Autodesk Fusion 360 part; units mm, degrees
(part 4 of 9)
  spline S95 degree 3 poles (-31.9349, 64.8889) (-32.1312, 64.9819) (-32.4392, 65.0284) (-32.8599, 65.0284) knots 0 0 0 0 1 1 1 1
  line L121 (-32.8599, 65.0284) -> (-35.2008, 65.0284)
  line L122 (-35.2008, 65.0284) -> (-35.2008, 61.7728)
  line L123 (-35.2008, 61.7728) -> (-36.2292, 61.7728)
  line L124 (-36.2292, 61.7728) -> (-36.2292, 69.3641)
  line L125 (-13.5711, 69.3641) -> (-13.5711, 68.4598)
  line L126 (-13.5711, 68.4598) -> (-16.1291, 68.4598)
  line L127 (-16.1291, 68.4598) -> (-16.1291, 61.7728)
  line L128 (-16.1291, 61.7728) -> (-17.173, 61.7728)
  line L129 (-17.173, 61.7728) -> (-17.173, 68.4598)
  line L130 (-17.173, 68.4598) -> (-19.7309, 68.4598)
  line L131 (-19.7309, 68.4598) -> (-19.7309, 69.3641)
  line L132 (-19.7309, 69.3641) -> (-13.5711, 69.3641)
  line L133 (-1.8995, 69.3641) -> (-1.8995, 64.6719)
  spline S96 degree 3 poles (-1.8995, 64.6719) (-1.8995, 64.121) (-1.7961, 63.6621) (-1.5894, 63.2973) knots 0 0 0 0 1 1 1 1
  spline S97 degree 3 poles (-1.5894, 63.2973) (-1.2825, 62.7464) (-0.7657, 62.4705) (-0.0391, 62.4705) knots 0 0 0 0 1 1 1 1
  spline S98 degree 3 poles (-0.0391, 62.4705) (0.8321, 62.4705) (1.4254, 62.7681) (1.7385, 63.3645) knots 0 0 0 0 1 1 1 1
  spline S99 degree 3 poles (1.7385, 63.3645) (1.907, 63.688) (1.9918, 64.1241) (1.9918, 64.6719) knots 0 0 0 0 1 1 1 1
  line L134 (1.9918, 64.6719) -> (1.9918, 69.3641)
  line L135 (1.9918, 69.3641) -> (3.0356, 69.3641)
  line L136 (3.0356, 69.3641) -> (3.0356, 65.1008)
  spline S100 degree 3 poles (3.0356, 65.1008) (3.0356, 64.1675) (2.9095, 63.4492) (2.6584, 62.9459) knots 0 0 0 0 1 1 1 1
  spline S101 degree 3 poles (2.6584, 62.9459) (2.1964, 62.0291) (1.3251, 61.5713) (0.0436, 61.5713) knots 0 0 0 0 1 1 1 1
  spline S102 degree 3 poles (0.0436, 61.5713) (-1.238, 61.5713) (-2.1083, 62.0291) (-2.5661, 62.9459) knots 0 0 0 0 1 1 1 1
  spline S103 degree 3 poles (-2.5661, 62.9459) (-2.8173, 63.4492) (-2.9433, 64.1675) (-2.9433, 65.1008) knots 0 0 0 0 1 1 1 1
  line L137 (-2.9433, 65.1008) -> (-2.9433, 69.3641)
  line L138 (-2.9433, 69.3641) -> (-1.8995, 69.3641)
  line L139 (13.6531, 69.3641) -> (14.8675, 69.3641)
  line L140 (14.8675, 69.3641) -> (18.7018, 63.2146)
  line L141 (18.7018, 63.2146) -> (18.7018, 69.3641)
  line L142 (18.7018, 69.3641) -> (19.6785, 69.3641)
  line L143 (19.6785, 69.3641) -> (19.6785, 61.7728)
  line L144 (19.6785, 61.7728) -> (18.5261, 61.7728)
  line L145 (18.5261, 61.7728) -> (14.6349, 67.9172)
  line L146 (14.6349, 67.9172) -> (14.6349, 61.7728)
  line L147 (14.6349, 61.7728) -> (13.6531, 61.7728)
  line L148 (13.6531, 61.7728) -> (13.6531, 69.3641)
  line L149 (31.0091, 69.3641) -> (36.2749, 69.3641)
  line L150 (36.2749, 69.3641) -> (36.2749, 68.4339)
  line L151 (36.2749, 68.4339) -> (32.0375, 68.4339)
  line L152 (32.0375, 68.4339) -> (32.0375, 66.1292)
  line L153 (32.0375, 66.1292) -> (35.7633, 66.1292)
  line L154 (35.7633, 66.1292) -> (35.7633, 65.2248)
  line L155 (35.7633, 65.2248) -> (32.0375, 65.2248)
  line L156 (32.0375, 65.2248) -> (32.0375, 61.7728)
  line L157 (32.0375, 61.7728) -> (31.0091, 61.7728)
  line L158 (31.0091, 61.7728) -> (31.0091, 69.3641)
  line L159 (47.0164, 62.6255) -> (51.6724, 68.4598)
  line L160 (51.6724, 68.4598) -> (47.3575, 68.4598)
  line L161 (47.3575, 68.4598) -> (47.3575, 69.3641)
  line L162 (47.3575, 69.3641) -> (52.9954, 69.3641)
  line L163 (52.9954, 69.3641) -> (52.9954, 68.4804)
  line L164 (52.9954, 68.4804) -> (48.3135, 62.6772)
  line L165 (48.3135, 62.6772) -> (52.9954, 62.6772)
  line L166 (52.9954, 62.6772) -> (52.9954, 61.7728)
  line L167 (52.9954, 61.7728) -> (47.0164, 61.7728)
  line L168 (47.0164, 61.7728) -> (47.0164, 62.6255)
  line L169 (67.8482, 64.8837) -> (66.6958, 68.2375)
  line L170 (66.6958, 68.2375) -> (65.4711, 64.8837)
  line L171 (65.4711, 64.8837) -> (67.8482, 64.8837)
  line L172 (66.1584, 69.3641) -> (67.3211, 69.3641)
  line L173 (67.3211, 69.3641) -> (70.0755, 61.7728)
  line L174 (70.0755, 61.7728) -> (68.9489, 61.7728)
  line L175 (68.9489, 61.7728) -> (68.1789, 64.0466)
  line L176 (68.1789, 64.0466) -> (65.1765, 64.0466)
  line L177 (65.1765, 64.0466) -> (64.3549, 61.7728)
  line L178 (64.3549, 61.7728) -> (63.3007, 61.7728)
  line L179 (63.3007, 61.7728) -> (66.1584, 69.3641)
  line L180 (67.0576, 71.1624) -> (68.0239, 71.1624)
  line L181 (68.0239, 71.1624) -> (68.0239, 70.0876)
  line L182 (68.0239, 70.0876) -> (67.0576, 70.0876)
  line L183 (67.0576, 70.0876) -> (67.0576, 71.1624)
  line L184 (65.3522, 71.1624) -> (66.3186, 71.1624)
  line L185 (66.3186, 71.1624) -> (66.3186, 70.0876)
  line L186 (66.3186, 70.0876) -> (65.3522, 70.0876)
  line L187 (65.3522, 70.0876) -> (65.3522, 71.1624)
  line L188 (84.517, 64.8837) -> (83.3646, 68.2375)
  line L189 (83.3646, 68.2375) -> (82.1398, 64.8837)
  line L190 (82.1398, 64.8837) -> (84.517, 64.8837)
  line L191 (82.8271, 69.3641) -> (83.9899, 69.3641)
  line L192 (83.9899, 69.3641) -> (86.7442, 61.7728)
  line L193 (86.7442, 61.7728) -> (85.6177, 61.7728)
  line L194 (85.6177, 61.7728) -> (84.8477, 64.0466)
  line L195 (84.8477, 64.0466) -> (81.8453, 64.0466)
  line L196 (81.8453, 64.0466) -> (81.0236, 61.7728)
  line L197 (81.0236, 61.7728) -> (79.9694, 61.7728)
  line L198 (79.9694, 61.7728) -> (82.8271, 69.3641)
  line L199 (83.7263, 71.1624) -> (84.6927, 71.1624)
  line L200 (84.6927, 71.1624) -> (84.6927, 70.0876)
  line L201 (84.6927, 70.0876) -> (83.7263, 70.0876)
  line L202 (83.7263, 70.0876) -> (83.7263, 71.1624)
  line L203 (82.021, 71.1624) -> (82.9873, 71.1624)
  line L204 (82.9873, 71.1624) -> (82.9873, 70.0876)
  line L205 (82.9873, 70.0876) -> (82.021, 70.0876)
  line L206 (82.021, 70.0876) -> (82.021, 71.1624)
  line L207 (-86.3336, 44.1253) -> (-81.6776, 49.9596)
  line L208 (-81.6776, 49.9596) -> (-85.9925, 49.9596)
  line L209 (-85.9925, 49.9596) -> (-85.9925, 50.8639)
  line L210 (-85.9925, 50.8639) -> (-80.3546, 50.8639)
  line L211 (-80.3546, 50.8639) -> (-80.3546, 49.9803)
  line L212 (-80.3546, 49.9803) -> (-85.0365, 44.177)
  line L213 (-85.0365, 44.177) -> (-80.3546, 44.177)
  line L214 (-80.3546, 44.177) -> (-80.3546, 43.2727)
  line L215 (-80.3546, 43.2727) -> (-86.3336, 43.2727)
  line L216 (-86.3336, 43.2727) -> (-86.3336, 44.1253)
  line L217 (-70.3615, 50.8639) -> (-68.93, 44.6886)
  line L218 (-68.93, 44.6886) -> (-67.2144, 50.8639)
  line L219 (-67.2144, 50.8639) -> (-66.0981, 50.8639)
  line L220 (-66.0981, 50.8639) -> (-64.3825, 44.6886)
  line L221 (-64.3825, 44.6886) -> (-62.951, 50.8639)
  line L222 (-62.951, 50.8639) -> (-61.8245, 50.8639)
  line L223 (-61.8245, 50.8639) -> (-63.8192, 43.2727)
  line L224 (-63.8192, 43.2727) -> (-64.8993, 43.2727)
  line L225 (-64.8993, 43.2727) -> (-66.6511, 49.5669)
  line L226 (-66.6511, 49.5669) -> (-68.4132, 43.2727)
  line L227 (-68.4132, 43.2727) -> (-69.4933, 43.2727)
  line L228 (-69.4933, 43.2727) -> (-71.4777, 50.8639)
  line L229 (-71.4777, 50.8639) -> (-70.3615, 50.8639)
  line L230 (-48.833, 46.3836) -> (-49.9854, 49.7374)
  line L231 (-49.9854, 49.7374) -> (-51.2102, 46.3836)
  line L232 (-51.2102, 46.3836) -> (-48.833, 46.3836)
  line L233 (-50.5229, 50.8639) -> (-49.3601, 50.8639)
  line L234 (-49.3601, 50.8639) -> (-46.6058, 43.2727)
  line L235 (-46.6058, 43.2727) -> (-47.7323, 43.2727)
  line L236 (-47.7323, 43.2727) -> (-48.5023, 45.5464)
  line L237 (-48.5023, 45.5464) -> (-51.5047, 45.5464)
  line L238 (-51.5047, 45.5464) -> (-52.3264, 43.2727)
  line L239 (-52.3264, 43.2727) -> (-53.3806, 43.2727)
  line L240 (-53.3806, 43.2727) -> (-50.5229, 50.8639)
  line L241 (-49.6237, 52.6623) -> (-48.6573, 52.6623)
  line L242 (-48.6573, 52.6623) -> (-48.6573, 51.5874)
  line L243 (-48.6573, 51.5874) -> (-49.6237, 51.5874)
  line L244 (-49.6237, 51.5874) -> (-49.6237, 52.6623)
  line L245 (-51.329, 52.6623) -> (-50.3627, 52.6623)
  line L246 (-50.3627, 52.6623) -> (-50.3627, 51.5874)
  line L247 (-50.3627, 51.5874) -> (-51.329, 51.5874)
  line L248 (-51.329, 51.5874) -> (-51.329, 52.6623)
  line L249 (-36.3532, 50.8639) -> (-35.1388, 50.8639)
  line L250 (-35.1388, 50.8639) -> (-31.3044, 44.7144)
  line L251 (-31.3044, 44.7144) -> (-31.3044, 50.8639)
  line L252 (-31.3044, 50.8639) -> (-30.3277, 50.8639)
  line L253 (-30.3277, 50.8639) -> (-30.3277, 43.2727)
  line L254 (-30.3277, 43.2727) -> (-31.4801, 43.2727)
  line L255 (-31.4801, 43.2727) -> (-35.3713, 49.417)
  line L256 (-35.3713, 49.417) -> (-35.3713, 43.2727)
  line L257 (-35.3713, 43.2727) -> (-36.3532, 43.2727)
  line L258 (-36.3532, 43.2727) -> (-36.3532, 50.8639)
  line L259 (-19.6586, 44.1253) -> (-15.0026, 49.9596)
  line L260 (-15.0026, 49.9596) -> (-19.3175, 49.9596)
  line L261 (-19.3175, 49.9596) -> (-19.3175, 50.8639)
  line L262 (-19.3175, 50.8639) -> (-13.6796, 50.8639)
  line L263 (-13.6796, 50.8639) -> (-13.6796, 49.9803)
  line L264 (-13.6796, 49.9803) -> (-18.3615, 44.177)
  line L265 (-18.3615, 44.177) -> (-13.6796, 44.177)
  line L266 (-13.6796, 44.177) -> (-13.6796, 43.2727)
  line L267 (-13.6796, 43.2727) -> (-19.6586, 43.2727)
  line L268 (-19.6586, 43.2727) -> (-19.6586, 44.1253)
  spline S104 degree 3 poles (-0.0278, 51.0603) (0.6854, 51.0603) (1.3024, 50.9228) (1.8223, 50.6469) knots 0 0 0 0 1 1 1 1
  spline S105 degree 3 poles (1.8223, 50.6469) (2.5767, 50.251) (3.0387, 49.5565) (3.2072, 48.5643) knots 0 0 0 0 1 1 1 1
  line L269 (3.2072, 48.5643) -> (2.1892, 48.5643)
  spline S106 degree 3 poles (2.1892, 48.5643) (2.0651, 49.1193) (1.8088, 49.5234) (1.4192, 49.7756) knots 0 0 0 0 1 1 1 1
  spline S107 degree 3 poles (1.4192, 49.7756) (1.0295, 50.0288) (0.5386, 50.156) (-0.0536, 50.156) knots 0 0 0 0 1 1 1 1
  spline S108 degree 3 poles (-0.0536, 50.156) (-0.7564, 50.156) (-1.3476, 49.8924) (-1.8292, 49.3653) knots 0 0 0 0 1 1 1 1
  spline S109 degree 3 poles (-1.8292, 49.3653) (-2.3098, 48.8382) (-2.5496, 48.0527) (-2.5496, 47.0089) knots 0 0 0 0 1 1 1 1
  spline S110 degree 3 poles (-2.5496, 47.0089) (-2.5496, 46.1066) (-2.3511, 45.3718) (-1.9553, 44.8044) knots 0 0 0 0 1 1 1 1
  spline S111 degree 3 poles (-1.9553, 44.8044) (-1.5594, 44.238) (-0.9135, 43.9548) (-0.0174, 43.9548) knots 0 0 0 0 1 1 1 1
  spline S112 degree 3 poles (-0.0174, 43.9548) (0.6678, 43.9548) (1.2362, 44.1532) (1.6848, 44.5522) knots 0 0 0 0 1 1 1 1
  spline S113 degree 3 poles (1.6848, 44.5522) (2.1344, 44.9501) (2.3649, 45.5929) (2.3752, 46.4818) knots 0 0 0 0 1 1 1 1
  line L270 (2.3752, 46.4818) -> (-0.0019, 46.4818)
  line L271 (-0.0019, 46.4818) -> (-0.0019, 47.3344)
  line L272 (-0.0019, 47.3344) -> (3.3312, 47.3344)
  line L273 (3.3312, 47.3344) -> (3.3312, 43.2727)
  line L274 (3.3312, 43.2727) -> (2.6698, 43.2727)
  line L275 (2.6698, 43.2727) -> (2.4217, 44.2493)
  spline S114 degree 3 poles (2.4217, 44.2493) (2.0734, 43.8669) (1.7654, 43.6013) (1.4967, 43.4535) knots 0 0 0 0 1 1 1 1
  spline S115 degree 3 poles (1.4967, 43.4535) (1.045, 43.1983) (0.4714, 43.0711) (-0.2241, 43.0711) knots 0 0 0 0 1 1 1 1
  spline S116 degree 3 poles (-0.2241, 43.0711) (-1.1233, 43.0711) (-1.8964, 43.3626) (-2.5444, 43.9445) knots 0 0 0 0 1 1 1 1
  spline S117 degree 3 poles (-2.5444, 43.9445) (-3.2503, 44.6752) (-3.6038, 45.6777) (-3.6038, 46.952) knots 0 0 0 0 1 1 1 1
  spline S118 degree 3 poles (-3.6038, 46.952) (-3.6038, 48.2233) (-3.2596, 49.2341) (-2.5702, 49.9854) knots 0 0 0 0 1 1 1 1
  spline S119 degree 3 poles (-2.5702, 49.9854) (-1.916, 50.7017) (-1.0685, 51.0603) (-0.0278, 51.0603) knots 0 0 0 0 1 1 1 1
  spline S120 degree 3 poles (14.6173, 45.7221) (14.6411, 45.2911) (14.7434, 44.9418) (14.9222, 44.6731) knots 0 0 0 0 1 1 1 1
  spline S121 degree 3 poles (14.9222, 44.6731) (15.2633, 44.1698) (15.8648, 43.9186) (16.7257, 43.9186) knots 0 0 0 0 1 1 1 1
  spline S122 degree 3 poles (16.7257, 43.9186) (17.1112, 43.9186) (17.4626, 43.9734) (17.7799, 44.084) knots 0 0 0 0 1 1 1 1
  spline S123 degree 3 poles (17.7799, 44.084) (18.3928, 44.2979) (18.6998, 44.6803) (18.6998, 45.2312) knots 0 0 0 0 1 1 1 1
  spline S124 degree 3 poles (18.6998, 45.2312) (18.6998, 45.6446) (18.5706, 45.9392) (18.3122, 46.1149) knots 0 0 0 0 1 1 1 1
  spline S125 degree 3 poles (18.3122, 46.1149) (18.0507, 46.2875) (17.6404, 46.4373) (17.0823, 46.5645) knots 0 0 0 0 1 1 1 1
  line L276 (17.0823, 46.5645) -> (16.0539, 46.797)
  spline S126 degree 3 poles (16.0539, 46.797) (15.3822, 46.9489) (14.9067, 47.1153) (14.6277, 47.2983) knots 0 0 0 0 1 1 1 1
  spline S127 degree 3 poles (14.6277, 47.2983) (14.145, 47.6156) (13.9042, 48.0889) (13.9042, 48.7194) knots 0 0 0 0 1 1 1 1
  spline S128 degree 3 poles (13.9042, 48.7194) (13.9042, 49.4015) (14.1399, 49.9617) (14.6122, 50.3988) knots 0 0 0 0 1 1 1 1
  spline S129 degree 3 poles (14.6122, 50.3988) (15.0845, 50.836) (15.7522, 51.0551) (16.6172, 51.0551) knots 0 0 0 0 1 1 1 1
  spline S130 degree 3 poles (16.6172, 51.0551) (17.413, 51.0551) (18.089, 50.8629) (18.646, 50.4784) knots 0 0 0 0 1 1 1 1
  spline S131 degree 3 poles (18.646, 50.4784) (19.2021, 50.095) (19.4801, 49.4811) (19.4801, 48.6367) knots 0 0 0 0 1 1 1 1
  line L277 (19.4801, 48.6367) -> (18.5137, 48.6367)
  spline S132 degree 3 poles (18.5137, 48.6367) (18.4621, 49.0429) (18.3515, 49.355) (18.183, 49.572) knots 0 0 0 0 1 1 1 1
  spline S133 degree 3 poles (18.183, 49.572) (17.8699, 49.9679) (17.3376, 50.1663) (16.5862, 50.1663) knots 0 0 0 0 1 1 1 1
  spline S134 degree 3 poles (16.5862, 50.1663) (15.9795, 50.1663) (15.5444, 50.0392) (15.2788, 49.7839) knots 0 0 0 0 1 1 1 1
  spline S135 degree 3 poles (15.2788, 49.7839) (15.0132, 49.5286) (14.8809, 49.233) (14.8809, 48.8951) knots 0 0 0 0 1 1 1 1
  spline S136 degree 3 poles (14.8809, 48.8951) (14.8809, 48.523) (15.0359, 48.2512) (15.346, 48.0786) knots 0 0 0 0 1 1 1 1
  spline S137 degree 3 poles (15.346, 48.0786) (15.5496, 47.968) (16.0095, 47.8305) (16.7257, 47.6652) knots 0 0 0 0 1 1 1 1
  line L278 (16.7257, 47.6652) -> (17.7903, 47.4223)
  spline S138 degree 3 poles (17.7903, 47.4223) (18.3039, 47.3055) (18.6998, 47.1453) (18.9788, 46.9417) knots 0 0 0 0 1 1 1 1
  spline S139 degree 3 poles (18.9788, 46.9417) (19.4615, 46.5872) (19.7023, 46.0715) (19.7023, 45.3966) knots 0 0 0 0 1 1 1 1
  spline S140 degree 3 poles (19.7023, 45.3966) (19.7023, 44.5563) (19.3964, 43.9548) (18.7845, 43.5931) knots 0 0 0 0 1 1 1 1
  spline S141 degree 3 poles (18.7845, 43.5931) (18.1737, 43.2313) (17.4626, 43.0505) (16.6534, 43.0505) knots 0 0 0 0 1 1 1 1
  spline S142 degree 3 poles (16.6534, 43.0505) (15.7098, 43.0505) (14.9708, 43.2913) (14.4365, 43.7739) knots 0 0 0 0 1 1 1 1
  spline S143 degree 3 poles (14.4365, 43.7739) (13.9021, 44.2524) (13.6407, 44.9025) (13.651, 45.7221) knots 0 0 0 0 1 1 1 1
  line L279 (13.651, 45.7221) -> (14.6173, 45.7221)
  line L280 (30.7125, 50.8639) -> (36.247, 50.8639)
  line L281 (36.247, 50.8639) -> (36.247, 49.9338)
  line L282 (36.247, 49.9338) -> (31.715, 49.9338)
  line L283 (31.715, 49.9338) -> (31.715, 47.629)
  line L284 (31.715, 47.629) -> (35.906, 47.629)
  line L285 (35.906, 47.629) -> (35.906, 46.7505)
  line L286 (35.906, 46.7505) -> (31.715, 46.7505)
  line L287 (31.715, 46.7505) -> (31.715, 44.177)
  line L288 (31.715, 44.177) -> (36.3245, 44.177)
  line L289 (36.3245, 44.177) -> (36.3245, 43.2727)
  line L290 (36.3245, 43.2727) -> (30.7125, 43.2727)
  line L291 (30.7125, 43.2727) -> (30.7125, 50.8639)
  line L292 (47.8825, 50.8639) -> (50.0632, 44.3992)
  line L293 (50.0632, 44.3992) -> (52.2181, 50.8639)
  line L294 (52.2181, 50.8639) -> (53.3705, 50.8639)
  line L295 (53.3705, 50.8639) -> (50.6007, 43.2727)
  line L296 (50.6007, 43.2727) -> (49.5103, 43.2727)
  line L297 (49.5103, 43.2727) -> (46.7456, 50.8639)
  line L298 (46.7456, 50.8639) -> (47.8825, 50.8639)
  spline S144 degree 3 poles (66.6421, 51.0706) (67.9826, 51.0706) (68.9747, 50.6397) (69.6186, 49.7787) knots 0 0 0 0 1 1 1 1
  spline S145 degree 3 poles (69.6186, 49.7787) (70.122, 49.1069) (70.3731, 48.247) (70.3731, 47.2001) knots 0 0 0 0 1 1 1 1
  spline S146 degree 3 poles (70.3731, 47.2001) (70.3731, 46.0663) (70.0858, 45.1247) (69.5101, 44.3734) knots 0 0 0 0 1 1 1 1
  spline S147 degree 3 poles (69.5101, 44.3734) (68.8352, 43.4918) (67.872, 43.0505) (66.6214, 43.0505) knots 0 0 0 0 1 1 1 1
  spline S148 degree 3 poles (66.6214, 43.0505) (65.4535, 43.0505) (64.5357, 43.436) (63.867, 44.208) knots 0 0 0 0 1 1 1 1
  spline S149 degree 3 poles (63.867, 44.208) (63.2707, 44.9521) (62.973, 45.8927) (62.973, 47.0295) knots 0 0 0 0 1 1 1 1
  spline S150 degree 3 poles (62.973, 47.0295) (62.973, 48.0558) (63.2283, 48.9343) (63.7379, 49.665) knots 0 0 0 0 1 1 1 1
  spline S151 degree 3 poles (63.7379, 49.665) (64.3921, 50.6024) (65.3605, 51.0706) (66.6421, 51.0706) knots 0 0 0 0 1 1 1 1
  spline S152 degree 3 poles (66.7454, 43.9703) (67.6518, 43.9703) (68.3071, 44.2948) (68.7112, 44.9449) knots 0 0 0 0 1 1 1 1
  spline S153 degree 3 poles (68.7112, 44.9449) (69.1163, 45.594) (69.3189, 46.3402) (69.3189, 47.1846) knots 0 0 0 0 1 1 1 1
  spline S154 degree 3 poles (69.3189, 47.1846) (69.3189, 48.0765) (69.0853, 48.7948) (68.6182, 49.3395) knots 0 0 0 0 1 1 1 1
  spline S155 degree 3 poles (68.6182, 49.3395) (68.1521, 49.8841) (67.5133, 50.156) (66.7041, 50.156) knots 0 0 0 0 1 1 1 1
  spline S156 degree 3 poles (66.7041, 50.156) (65.9186, 50.156) (65.2778, 49.8862) (64.7817, 49.3477) knots 0 0 0 0 1 1 1 1
  spline S157 degree 3 poles (64.7817, 49.3477) (64.2856, 48.8082) (64.0376, 48.0135) (64.0376, 46.9624) knots 0 0 0 0 1 1 1 1
  spline S158 degree 3 poles (64.0376, 46.9624) (64.0376, 46.1221) (64.2505, 45.4131) (64.6763, 44.8354) knots 0 0 0 0 1 1 1 1
  spline S159 degree 3 poles (64.6763, 44.8354) (65.1011, 44.2587) (65.7915, 43.9703) (66.7454, 43.9703) knots 0 0 0 0 1 1 1 1
  spline S160 degree 3 poles (83.8576, 47.3861) (84.3402, 47.3861) (84.7216, 47.4822) (85.0017, 47.6755) knots 0 0 0 0 1 1 1 1
  spline S161 degree 3 poles (85.0017, 47.6755) (85.2828, 47.8688) (85.4234, 48.216) (85.4234, 48.7194) knots 0 0 0 0 1 1 1 1
  spline S162 degree 3 poles (85.4234, 48.7194) (85.4234, 49.2599) (85.227, 49.6289) (84.8342, 49.8252) knots 0 0 0 0 1 1 1 1
  spline S163 degree 3 poles (84.8342, 49.8252) (84.6244, 49.9286) (84.3433, 49.9803) (83.9919, 49.9803) knots 0 0 0 0 1 1 1 1
  line L299 (83.9919, 49.9803) -> (81.4804, 49.9803)
  line L300 (81.4804, 49.9803) -> (81.4804, 47.3861)
  line L301 (81.4804, 47.3861) -> (83.8576, 47.3861)
  line L302 (80.4521, 50.8639) -> (83.9661, 50.8639)
  spline S164 degree 3 poles (83.9661, 50.8639) (84.5449, 50.8639) (85.0223, 50.7792) (85.3975, 50.6107) knots 0 0 0 0 1 1 1 1
  spline S165 degree 3 poles (85.3975, 50.6107) (86.1107, 50.2872) (86.4672, 49.6888) (86.4672, 48.8175) knots 0 0 0 0 1 1 1 1
  spline S166 degree 3 poles (86.4672, 48.8175) (86.4672, 48.3628) (86.3732, 47.9907) (86.1861, 47.7013) knots 0 0 0 0 1 1 1 1
  spline S167 degree 3 poles (86.1861, 47.7013) (85.998, 47.4119) (85.7355, 47.1794) (85.3975, 47.0037) knots 0 0 0 0 1 1 1 1
  spline S168 degree 3 poles (85.3975, 47.0037) (85.6941, 46.8828) (85.9174, 46.7247) (86.0662, 46.5283) knots 0 0 0 0 1 1 1 1
  spline S169 degree 3 poles (86.0662, 46.5283) (86.2161, 46.3319) (86.2998, 46.0136) (86.3174, 45.5723) knots 0 0 0 0 1 1 1 1
  line L303 (86.3174, 45.5723) -> (86.3535, 44.5542)
  spline S170 degree 3 poles (86.3535, 44.5542) (86.3639, 44.2649) (86.3876, 44.0499) (86.4259, 43.9083) knots 0 0 0 0 1 1 1 1
  spline S171 degree 3 poles (86.4259, 43.9083) (86.4879, 43.6675) (86.5985, 43.5124) (86.7566, 43.4432) knots 0 0 0 0 1 1 1 1
  line L304 (86.7566, 43.4432) -> (86.7566, 43.2727)
  line L305 (86.7566, 43.2727) -> (85.4957, 43.2727)
  spline S172 degree 3 poles (85.4957, 43.2727) (85.4616, 43.3378) (85.4337, 43.4225) (85.413, 43.5259) knots 0 0 0 0 1 1 1 1
  spline S173 degree 3 poles (85.413, 43.5259) (85.3924, 43.6292) (85.3748, 43.8287) (85.3613, 44.1253) knots 0 0 0 0 1 1 1 1
  line L306 (85.3613, 44.1253) -> (85.2993, 45.3914)
  spline S174 degree 3 poles (85.2993, 45.3914) (85.2756, 45.8875) (85.0906, 46.2203) (84.7464, 46.3888) knots 0 0 0 0 1 1 1 1
  spline S175 degree 3 poles (84.7464, 46.3888) (84.55, 46.4818) (84.242, 46.5283) (83.8214, 46.5283) knots 0 0 0 0 1 1 1 1
  line L307 (83.8214, 46.5283) -> (81.4804, 46.5283)
  line L308 (81.4804, 46.5283) -> (81.4804, 43.2727)
  line L309 (81.4804, 43.2727) -> (80.4521, 43.2727)
  line L310 (80.4521, 43.2727) -> (80.4521, 50.8639)
  line L311 (-82.1705, 27.8834) -> (-83.3229, 31.2372)
  line L312 (-83.3229, 31.2372) -> (-84.5477, 27.8834)
  line L313 (-84.5477, 27.8834) -> (-82.1705, 27.8834)
  line L314 (-83.8604, 32.3638) -> (-82.6976, 32.3638)
  line L315 (-82.6976, 32.3638) -> (-79.9433, 24.7725)
  line L316 (-79.9433, 24.7725) -> (-81.0698, 24.7725)
  line L317 (-81.0698, 24.7725) -> (-81.8398, 27.0463)
  line L318 (-81.8398, 27.0463) -> (-84.8422, 27.0463)
  line L319 (-84.8422, 27.0463) -> (-85.6639, 24.7725)
  line L320 (-85.6639, 24.7725) -> (-86.7181, 24.7725)
  line L321 (-86.7181, 24.7725) -> (-83.8604, 32.3638)
  spline S176 degree 3 poles (-66.5457, 29.1547) (-66.1116, 29.1547) (-65.7736, 29.2146) (-65.5328, 29.3355) knots 0 0 0 0 1 1 1 1
  spline S177 degree 3 poles (-65.5328, 29.3355) (-65.1535, 29.5247) (-64.9644, 29.8657) (-64.9644, 30.3587) knots 0 0 0 0 1 1 1 1
  spline S178 degree 3 poles (-64.9644, 30.3587) (-64.9644, 30.8548) (-65.1659, 31.1886) (-65.569, 31.3612) knots 0 0 0 0 1 1 1 1
  spline S179 degree 3 poles (-65.569, 31.3612) (-65.7964, 31.4574) (-66.1343, 31.5059) (-66.5818, 31.5059) knots 0 0 0 0 1 1 1 1
  line L322 (-66.5818, 31.5059) -> (-68.4163, 31.5059)
  line L323 (-68.4163, 31.5059) -> (-68.4163, 29.1547)
  line L324 (-68.4163, 29.1547) -> (-66.5457, 29.1547)
  spline S180 degree 3 poles (-66.1994, 25.651) (-65.569, 25.651) (-65.1194, 25.8339) (-64.8507, 26.1988) knots 0 0 0 0 1 1 1 1
  spline S181 degree 3 poles (-64.8507, 26.1988) (-64.6822, 26.4292) (-64.5975, 26.7083) (-64.5975, 27.0359) knots 0 0 0 0 1 1 1 1
  spline S182 degree 3 poles (-64.5975, 27.0359) (-64.5975, 27.5868) (-64.8434, 27.963) (-65.3364, 28.1625) knots 0 0 0 0 1 1 1 1
  spline S183 degree 3 poles (-65.3364, 28.1625) (-65.5979, 28.2689) (-65.9441, 28.3227) (-66.3751, 28.3227) knots 0 0 0 0 1 1 1 1
  line L325 (-66.3751, 28.3227) -> (-68.4163, 28.3227)
  line L326 (-68.4163, 28.3227) -> (-68.4163, 25.651)
  line L327 (-68.4163, 25.651) -> (-66.1994, 25.651)
  line L328 (-69.424, 32.3638) -> (-66.1633, 32.3638)
  spline S184 degree 3 poles (-66.1633, 32.3638) (-65.2744, 32.3638) (-64.6419, 32.0982) (-64.2667, 31.568) knots 0 0 0 0 1 1 1 1
  spline S185 degree 3 poles (-64.2667, 31.568) (-64.0466, 31.2548) (-63.936, 30.8931) (-63.936, 30.4827) knots 0 0 0 0 1 1 1 1
  spline S186 degree 3 poles (-63.936, 30.4827) (-63.936, 30.0042) (-64.0724, 29.6115) (-64.3442, 29.3045) knots 0 0 0 0 1 1 1 1
  spline S187 degree 3 poles (-64.3442, 29.3045) (-64.4858, 29.1423) (-64.6884, 28.9945) (-64.954, 28.8601) knots 0 0 0 0 1 1 1 1
  spline S188 degree 3 poles (-64.954, 28.8601) (-64.5644, 28.7123) (-64.274, 28.5449) (-64.0807, 28.3588) knots 0 0 0 0 1 1 1 1
  spline S189 degree 3 poles (-64.0807, 28.3588) (-63.7396, 28.0281) (-63.5691, 27.5713) (-63.5691, 26.9894) knots 0 0 0 0 1 1 1 1
  spline S190 degree 3 poles (-63.5691, 26.9894) (-63.5691, 26.5006) (-63.7221, 26.0572) (-64.029, 25.6613) knots 0 0 0 0 1 1 1 1
  spline S191 degree 3 poles (-64.029, 25.6613) (-64.4869, 25.0691) (-65.2155, 24.7725) (-66.2149, 24.7725) knots 0 0 0 0 1 1 1 1
  line L329 (-66.2149, 24.7725) -> (-69.424, 24.7725)
  line L330 (-69.424, 24.7725) -> (-69.424, 32.3638)
  spline S192 degree 3 poles (-49.8232, 32.5705) (-48.862, 32.5705) (-48.1158, 32.3173) (-47.5856, 31.8108) knots 0 0 0 0 1 1 1 1
  spline S193 degree 3 poles (-47.5856, 31.8108) (-47.0554, 31.3044) (-46.7608, 30.7287) (-46.7019, 30.0848) knots 0 0 0 0 1 1 1 1
  line L331 (-46.7019, 30.0848) -> (-47.7044, 30.0848)
  spline S194 degree 3 poles (-47.7044, 30.0848) (-47.8181, 30.5737) (-48.0445, 30.9613) (-48.3835, 31.2476) knots 0 0 0 0 1 1 1 1
  spline S195 degree 3 poles (-48.3835, 31.2476) (-48.7235, 31.5338) (-49.2, 31.6765) (-49.8128, 31.6765) knots 0 0 0 0 1 1 1 1
  spline S196 degree 3 poles (-49.8128, 31.6765) (-50.5601, 31.6765) (-51.1637, 31.414) (-51.6246, 30.8889) knots 0 0 0 0 1 1 1 1
  spline S197 degree 3 poles (-51.6246, 30.8889) (-52.0845, 30.3629) (-52.314, 29.5577) (-52.314, 28.4725) knots 0 0 0 0 1 1 1 1
  spline S198 degree 3 poles (-52.314, 28.4725) (-52.314, 27.5837) (-52.1062, 26.8623) (-51.6908, 26.3104) knots 0 0 0 0 1 1 1 1
  spline S199 degree 3 poles (-51.6908, 26.3104) (-51.2763, 25.7575) (-50.6572, 25.4805) (-49.8335, 25.4805) knots 0 0 0 0 1 1 1 1
  spline S200 degree 3 poles (-49.8335, 25.4805) (-49.0759, 25.4805) (-48.4982, 25.7719) (-48.1023, 26.3538) knots 0 0 0 0 1 1 1 1
  spline S201 degree 3 poles (-48.1023, 26.3538) (-47.8925, 26.6608) (-47.7354, 27.0638) (-47.6321, 27.563) knots 0 0 0 0 1 1 1 1
  line L332 (-47.6321, 27.563) -> (-46.6296, 27.563)
  spline S202 degree 3 poles (-46.6296, 27.563) (-46.7195, 26.7641) (-47.0151, 26.0934) (-47.5184, 25.5528) knots 0 0 0 0 1 1 1 1
  spline S203 degree 3 poles (-47.5184, 25.5528) (-48.1209, 24.9017) (-48.9343, 24.5761) (-49.9575, 24.5761) knots 0 0 0 0 1 1 1 1
  spline S204 degree 3 poles (-49.9575, 24.5761) (-50.8391, 24.5761) (-51.5802, 24.8428) (-52.1796, 25.3771) knots 0 0 0 0 1 1 1 1
  spline S205 degree 3 poles (-52.1796, 25.3771) (-52.9682, 26.083) (-53.363, 27.1734) (-53.363, 28.6482) knots 0 0 0 0 1 1 1 1
  spline S206 degree 3 poles (-53.363, 28.6482) (-53.363, 29.7675) (-53.0664, 30.6864) (-52.4742, 31.4026) knots 0 0 0 0 1 1 1 1
  spline S207 degree 3 poles (-52.4742, 31.4026) (-51.8334, 32.1808) (-50.9497, 32.5705) (-49.8232, 32.5705) knots 0 0 0 0 1 1 1 1
  line L333 (-36.3274, 32.3638) -> (-35.2887, 32.3638)
  line L334 (-35.2887, 32.3638) -> (-35.2887, 29.227)
  line L335 (-35.2887, 29.227) -> (-31.3406, 29.227)
  line L336 (-31.3406, 29.227) -> (-31.3406, 32.3638)
  line L337 (-31.3406, 32.3638) -> (-30.3019, 32.3638)
  line L338 (-30.3019, 32.3638) -> (-30.3019, 24.7725)
  line L339 (-30.3019, 24.7725) -> (-31.3406, 24.7725)
  line L340 (-31.3406, 24.7725) -> (-31.3406, 28.3227)
  line L341 (-31.3406, 28.3227) -> (-35.2887, 28.3227)
  line L342 (-35.2887, 28.3227) -> (-35.2887, 24.7725)
  line L343 (-35.2887, 24.7725) -> (-36.3274, 24.7725)
  line L344 (-36.3274, 24.7725) -> (-36.3274, 32.3638)
  line L345 (-15.4955, 27.8834) -> (-16.6479, 31.2372)
  line L346 (-16.6479, 31.2372) -> (-17.8727, 27.8834)
  line L347 (-17.8727, 27.8834) -> (-15.4955, 27.8834)
  line L348 (-17.1854, 32.3638) -> (-16.0226, 32.3638)
  line L349 (-16.0226, 32.3638) -> (-13.2683, 24.7725)
  line L350 (-13.2683, 24.7725) -> (-14.3948, 24.7725)
  line L351 (-14.3948, 24.7725) -> (-15.1648, 27.0463)
  line L352 (-15.1648, 27.0463) -> (-18.1672, 27.0463)
  line L353 (-18.1672, 27.0463) -> (-18.9889, 24.7725)
  line L354 (-18.9889, 24.7725) -> (-20.0431, 24.7725)
  line L355 (-20.0431, 24.7725) -> (-17.1854, 32.3638)
  line L356 (-1.8995, 32.3638) -> (-1.8995, 27.6715)
  spline S208 degree 3 poles (-1.8995, 27.6715) (-1.8995, 27.1207) (-1.7961, 26.6618) (-1.5894, 26.297) knots 0 0 0 0 1 1 1 1
  spline S209 degree 3 poles (-1.5894, 26.297) (-1.2825, 25.7461) (-0.7657, 25.4701) (-0.0391, 25.4701) knots 0 0 0 0 1 1 1 1
  spline S210 degree 3 poles (-0.0391, 25.4701) (0.8321, 25.4701) (1.4254, 25.7678) (1.7385, 26.3641) knots 0 0 0 0 1 1 1 1
  spline S211 degree 3 poles (1.7385, 26.3641) (1.907, 26.6876) (1.9918, 27.1238) (1.9918, 27.6715) knots 0 0 0 0 1 1 1 1
  line L357 (1.9918, 27.6715) -> (1.9918, 32.3638)
  line L358 (1.9918, 32.3638) -> (3.0356, 32.3638)
  line L359 (3.0356, 32.3638) -> (3.0356, 28.1005)
  spline S212 degree 3 poles (3.0356, 28.1005) (3.0356, 27.1672) (2.9095, 26.4489) (2.6584, 25.9456) knots 0 0 0 0 1 1 1 1
  spline S213 degree 3 poles (2.6584, 25.9456) (2.1964, 25.0288) (1.3251, 24.571) (0.0436, 24.571) knots 0 0 0 0 1 1 1 1
  spline S214 degree 3 poles (0.0436, 24.571) (-1.238, 24.571) (-2.1083, 25.0288) (-2.5661, 25.9456) knots 0 0 0 0 1 1 1 1
  spline S215 degree 3 poles (-2.5661, 25.9456) (-2.8173, 26.4489) (-2.9433, 27.1672) (-2.9433, 28.1005) knots 0 0 0 0 1 1 1 1
  line L360 (-2.9433, 28.1005) -> (-2.9433, 32.3638)
  line L361 (-2.9433, 32.3638) -> (-1.8995, 32.3638)
  spline S216 degree 3 poles (16.7981, 29.1547) (17.2322, 29.1547) (17.5701, 29.2146) (17.8109, 29.3355) knots 0 0 0 0 1 1 1 1
  spline S217 degree 3 poles (17.8109, 29.3355) (18.1903, 29.5247) (18.3794, 29.8657) (18.3794, 30.3587) knots 0 0 0 0 1 1 1 1
  spline S218 degree 3 poles (18.3794, 30.3587) (18.3794, 30.8548) (18.1778, 31.1886) (17.7748, 31.3612) knots 0 0 0 0 1 1 1 1
  spline S219 degree 3 poles (17.7748, 31.3612) (17.5474, 31.4574) (17.2094, 31.5059) (16.7619, 31.5059) knots 0 0 0 0 1 1 1 1
  line L362 (16.7619, 31.5059) -> (14.9274, 31.5059)
  line L363 (14.9274, 31.5059) -> (14.9274, 29.1547)
  line L364 (14.9274, 29.1547) -> (16.7981, 29.1547)
  spline S220 degree 3 poles (17.1443, 25.651) (17.7748, 25.651) (18.2244, 25.8339) (18.4931, 26.1988) knots 0 0 0 0 1 1 1 1
  spline S221 degree 3 poles (18.4931, 26.1988) (18.6615, 26.4292) (18.7463, 26.7083) (18.7463, 27.0359) knots 0 0 0 0 1 1 1 1
  spline S222 degree 3 poles (18.7463, 27.0359) (18.7463, 27.5868) (18.5003, 27.963) (18.0073, 28.1625) knots 0 0 0 0 1 1 1 1
  spline S223 degree 3 poles (18.0073, 28.1625) (17.7458, 28.2689) (17.3996, 28.3227) (16.9686, 28.3227) knots 0 0 0 0 1 1 1 1
  line L365 (16.9686, 28.3227) -> (14.9274, 28.3227)
  line L366 (14.9274, 28.3227) -> (14.9274, 25.651)
  line L367 (14.9274, 25.651) -> (17.1443, 25.651)
  line L368 (13.9197, 32.3638) -> (17.1805, 32.3638)
  spline S224 degree 3 poles (17.1805, 32.3638) (18.0693, 32.3638) (18.7018, 32.0982) (19.077, 31.568) knots 0 0 0 0 1 1 1 1
  spline S225 degree 3 poles (19.077, 31.568) (19.2972, 31.2548) (19.4077, 30.8931) (19.4077, 30.4827) knots 0 0 0 0 1 1 1 1
  spline S226 degree 3 poles (19.4077, 30.4827) (19.4077, 30.0042) (19.2713, 29.6115) (18.9995, 29.3045) knots 0 0 0 0 1 1 1 1
  spline S227 degree 3 poles (18.9995, 29.3045) (18.8579, 29.1423) (18.6553, 28.9945) (18.3897, 28.8601) knots 0 0 0 0 1 1 1 1
  spline S228 degree 3 poles (18.3897, 28.8601) (18.7794, 28.7123) (19.0698, 28.5449) (19.2631, 28.3588) knots 0 0 0 0 1 1 1 1
  spline S229 degree 3 poles (19.2631, 28.3588) (19.6041, 28.0281) (19.7747, 27.5713) (19.7747, 26.9894) knots 0 0 0 0 1 1 1 1
  spline S230 degree 3 poles (19.7747, 26.9894) (19.7747, 26.5006) (19.6217, 26.0572) (19.3147, 25.6613) knots 0 0 0 0 1 1 1 1
  spline S231 degree 3 poles (19.3147, 25.6613) (18.8569, 25.0691) (18.1282, 24.7725) (17.1288, 24.7725) knots 0 0 0 0 1 1 1 1
  line L369 (17.1288, 24.7725) -> (13.9197, 24.7725)
  line L370 (13.9197, 24.7725) -> (13.9197, 32.3638)
  line L371 (32.9067, 32.3638) -> (33.9454, 32.3638)
  line L372 (33.9454, 32.3638) -> (33.9454, 24.7725)
  line L373 (33.9454, 24.7725) -> (32.9067, 24.7725)
  line L374 (32.9067, 24.7725) -> (32.9067, 32.3638)
  line L375 (47.3812, 32.3638) -> (52.9158, 32.3638)
  line L376 (52.9158, 32.3638) -> (52.9158, 31.4336)
  line L377 (52.9158, 31.4336) -> (48.3838, 31.4336)
  line L378 (48.3838, 31.4336) -> (48.3838, 29.1288)
  line L379 (48.3838, 29.1288) -> (52.5747, 29.1288)
  line L380 (52.5747, 29.1288) -> (52.5747, 28.2503)
  line L381 (52.5747, 28.2503) -> (48.3838, 28.2503)
  line L382 (48.3838, 28.2503) -> (48.3838, 25.6768)
  line L383 (48.3838, 25.6768) -> (52.9933, 25.6768)
  line L384 (52.9933, 25.6768) -> (52.9933, 24.7725)
  line L385 (52.9933, 24.7725) -> (47.3812, 24.7725)
  line L386 (47.3812, 24.7725) -> (47.3812, 32.3638)
  spline S232 degree 3 poles (66.8581, 32.5705) (67.8193, 32.5705) (68.5655, 32.3173) (69.0957, 31.8108) knots 0 0 0 0 1 1 1 1
  spline S233 degree 3 poles (69.0957, 31.8108) (69.6259, 31.3044) (69.9204, 30.7287) (69.9793, 30.0848) knots 0 0 0 0 1 1 1 1
  line L387 (69.9793, 30.0848) -> (68.9768, 30.0848)
  spline S234 degree 3 poles (68.9768, 30.0848) (68.8631, 30.5737) (68.6368, 30.9613) (68.2978, 31.2476) knots 0 0 0 0 1 1 1 1
  spline S235 degree 3 poles (68.2978, 31.2476) (67.9578, 31.5338) (67.4813, 31.6765) (66.8684, 31.6765) knots 0 0 0 0 1 1 1 1
  spline S236 degree 3 poles (66.8684, 31.6765) (66.1212, 31.6765) (65.5176, 31.414) (65.0566, 30.8889) knots 0 0 0 0 1 1 1 1
  spline S237 degree 3 poles (65.0566, 30.8889) (64.5967, 30.3629) (64.3673, 29.5577) (64.3673, 28.4725) knots 0 0 0 0 1 1 1 1
  spline S238 degree 3 poles (64.3673, 28.4725) (64.3673, 27.5837) (64.575, 26.8623) (64.9905, 26.3104) knots 0 0 0 0 1 1 1 1
  spline S239 degree 3 poles (64.9905, 26.3104) (65.4049, 25.7575) (66.024, 25.4805) (66.8477, 25.4805) knots 0 0 0 0 1 1 1 1
  spline S240 degree 3 poles (66.8477, 25.4805) (67.6053, 25.4805) (68.1831, 25.7719) (68.5789, 26.3538) knots 0 0 0 0 1 1 1 1
  spline S241 degree 3 poles (68.5789, 26.3538) (68.7887, 26.6608) (68.9458, 27.0638) (69.0492, 27.563) knots 0 0 0 0 1 1 1 1
  line L388 (69.0492, 27.563) -> (70.0517, 27.563)
  spline S242 degree 3 poles (70.0517, 27.563) (69.9618, 26.7641) (69.6662, 26.0934) (69.1628, 25.5528) knots 0 0 0 0 1 1 1 1
  spline S243 degree 3 poles (69.1628, 25.5528) (68.5603, 24.9017) (67.7469, 24.5761) (66.7237, 24.5761) knots 0 0 0 0 1 1 1 1
  spline S244 degree 3 poles (66.7237, 24.5761) (65.8421, 24.5761) (65.1011, 24.8428) (64.5016, 25.3771) knots 0 0 0 0 1 1 1 1
  spline S245 degree 3 poles (64.5016, 25.3771) (63.7131, 26.083) (63.3182, 27.1734) (63.3182, 28.6482) knots 0 0 0 0 1 1 1 1
  spline S246 degree 3 poles (63.3182, 28.6482) (63.3182, 29.7675) (63.6149, 30.6864) (64.2071, 31.4026) knots 0 0 0 0 1 1 1 1
  spline S247 degree 3 poles (64.2071, 31.4026) (64.8479, 32.1808) (65.7315, 32.5705) (66.8581, 32.5705) knots 0 0 0 0 1 1 1 1
  line L389 (79.7162, 32.3638) -> (81.189, 32.3638)
  line L390 (81.189, 32.3638) -> (83.3697, 25.9456)
  line L391 (83.3697, 25.9456) -> (85.535, 32.3638)
  line L392 (85.535, 32.3638) -> (86.9923, 32.3638)
  line L393 (86.9923, 32.3638) -> (86.9923, 24.7725)
  line L394 (86.9923, 24.7725) -> (86.0156, 24.7725)
  line L395 (86.0156, 24.7725) -> (86.0156, 29.2528)
  spline S248 degree 3 poles (86.0156, 29.2528) (86.0156, 29.4079) (86.0187, 29.6642) (86.0259, 30.0228) knots 0 0 0 0 1 1 1 1
  spline S249 degree 3 poles (86.0259, 30.0228) (86.0331, 30.3815) (86.0362, 30.7649) (86.0362, 31.1752) knots 0 0 0 0 1 1 1 1
  line L396 (86.0362, 31.1752) -> (83.871, 24.7725)
  line L397 (83.871, 24.7725) -> (82.853, 24.7725)
  line L398 (82.853, 24.7725) -> (80.6722, 31.1752)
  line L399 (80.6722, 31.1752) -> (80.6722, 30.9427)
  spline S250 degree 3 poles (80.6722, 30.9427) (80.6722, 30.7566) (80.6764, 30.4734) (80.6846, 30.0931) knots 0 0 0 0 1 1 1 1
  spline S251 degree 3 poles (80.6846, 30.0931) (80.6939, 29.7117) (80.6981, 29.4316) (80.6981, 29.2528) knots 0 0 0 0 1 1 1 1
  line L400 (80.6981, 29.2528) -> (80.6981, 24.7725)
  line L401 (80.6981, 24.7725) -> (79.7162, 24.7725)
  line L402 (79.7162, 24.7725) -> (79.7162, 32.3638)
  line L403 (-85.9688, 13.8636) -> (-80.4342, 13.8636)
  line L404 (-80.4342, 13.8636) -> (-80.4342, 12.9334)
  line L405 (-80.4342, 12.9334) -> (-84.9662, 12.9334)
  line L406 (-84.9662, 12.9334) -> (-84.9662, 10.6287)
  line L407 (-84.9662, 10.6287) -> (-80.7753, 10.6287)
  line L408 (-80.7753, 10.6287) -> (-80.7753, 9.7502)
  line L409 (-80.7753, 9.7502) -> (-84.9662, 9.7502)
  line L410 (-84.9662, 9.7502) -> (-84.9662, 7.1767)
  line L411 (-84.9662, 7.1767) -> (-80.3567, 7.1767)
  line L412 (-80.3567, 7.1767) -> (-80.3567, 6.2723)
  line L413 (-80.3567, 6.2723) -> (-85.9688, 6.2723)
  line L414 (-85.9688, 6.2723) -> (-85.9688, 13.8636)
  line L415 (-67.1058, 13.8636) -> (-66.0671, 13.8636)
  line L416 (-66.0671, 13.8636) -> (-66.0671, 6.2723)
  line L417 (-66.0671, 6.2723) -> (-67.1058, 6.2723)
  line L418 (-67.1058, 6.2723) -> (-67.1058, 13.8636)
  spline S252 degree 3 poles (-52.0577, 8.7218) (-52.0339, 8.2908) (-51.9316, 7.9415) (-51.7528, 7.6728) knots 0 0 0 0 1 1 1 1
  spline S253 degree 3 poles (-51.7528, 7.6728) (-51.4117, 7.1694) (-50.8102, 6.9183) (-49.9493, 6.9183) knots 0 0 0 0 1 1 1 1
  spline S254 degree 3 poles (-49.9493, 6.9183) (-49.5638, 6.9183) (-49.2124, 6.9731) (-48.8951, 7.0837) knots 0 0 0 0 1 1 1 1
  spline S255 degree 3 poles (-48.8951, 7.0837) (-48.2822, 7.2976) (-47.9752, 7.68) (-47.9752, 8.2309) knots 0 0 0 0 1 1 1 1
  spline S256 degree 3 poles (-47.9752, 8.2309) (-47.9752, 8.6443) (-48.1044, 8.9388) (-48.3628, 9.1145) knots 0 0 0 0 1 1 1 1
  spline S257 degree 3 poles (-48.3628, 9.1145) (-48.6243, 9.2871) (-49.0346, 9.437) (-49.5927, 9.5641) knots 0 0 0 0 1 1 1 1
  line L419 (-49.5927, 9.5641) -> (-50.6211, 9.7967)
  spline S258 degree 3 poles (-50.6211, 9.7967) (-51.2928, 9.9486) (-51.7683, 10.115) (-52.0473, 10.2979) knots 0 0 0 0 1 1 1 1
  spline S259 degree 3 poles (-52.0473, 10.2979) (-52.53, 10.6152) (-52.7708, 11.0886) (-52.7708, 11.719) knots 0 0 0 0 1 1 1 1
  spline S260 degree 3 poles (-52.7708, 11.719) (-52.7708, 12.4012) (-52.5351, 12.9613) (-52.0628, 13.3985) knots 0 0 0 0 1 1 1 1
  spline S261 degree 3 poles (-52.0628, 13.3985) (-51.5905, 13.8357) (-50.9228, 14.0548) (-50.0578, 14.0548) knots 0 0 0 0 1 1 1 1
  spline S262 degree 3 poles (-50.0578, 14.0548) (-49.262, 14.0548) (-48.586, 13.8626) (-48.029, 13.4781) knots 0 0 0 0 1 1 1 1
  spline S263 degree 3 poles (-48.029, 13.4781) (-47.4729, 13.0947) (-47.1949, 12.4807) (-47.1949, 11.6364) knots 0 0 0 0 1 1 1 1
  line L420 (-47.1949, 11.6364) -> (-48.1613, 11.6364)
  spline S264 degree 3 poles (-48.1613, 11.6364) (-48.2129, 12.0425) (-48.3235, 12.3547) (-48.492, 12.5717) knots 0 0 0 0 1 1 1 1
  spline S265 degree 3 poles (-48.492, 12.5717) (-48.8051, 12.9675) (-49.3374, 13.166) (-50.0888, 13.166) knots 0 0 0 0 1 1 1 1
  spline S266 degree 3 poles (-50.0888, 13.166) (-50.6955, 13.166) (-51.1306, 13.0389) (-51.3962, 12.7836) knots 0 0 0 0 1 1 1 1
  spline S267 degree 3 poles (-51.3962, 12.7836) (-51.6618, 12.5283) (-51.7941, 12.2327) (-51.7941, 11.8947) knots 0 0 0 0 1 1 1 1
  spline S268 degree 3 poles (-51.7941, 11.8947) (-51.7941, 11.5227) (-51.6391, 11.2508) (-51.329, 11.0782) knots 0 0 0 0 1 1 1 1
  spline S269 degree 3 poles (-51.329, 11.0782) (-51.1254, 10.9677) (-50.6655, 10.8302) (-49.9493, 10.6648) knots 0 0 0 0 1 1 1 1
  line L421 (-49.9493, 10.6648) -> (-48.8847, 10.422)
  spline S270 degree 3 poles (-48.8847, 10.422) (-48.3711, 10.3052) (-47.9752, 10.145) (-47.6962, 9.9414) knots 0 0 0 0 1 1 1 1
  spline S271 degree 3 poles (-47.6962, 9.9414) (-47.2135, 9.5869) (-46.9727, 9.0711) (-46.9727, 8.3962) knots 0 0 0 0 1 1 1 1
  spline S272 degree 3 poles (-46.9727, 8.3962) (-46.9727, 7.556) (-47.2786, 6.9545) (-47.8905, 6.5927) knots 0 0 0 0 1 1 1 1
  spline S273 degree 3 poles (-47.8905, 6.5927) (-48.5013, 6.231) (-49.2124, 6.0501) (-50.0216, 6.0501) knots 0 0 0 0 1 1 1 1
  spline S274 degree 3 poles (-50.0216, 6.0501) (-50.9652, 6.0501) (-51.7042, 6.2909) (-52.2385, 6.7736) knots 0 0 0 0 1 1 1 1
  spline S275 degree 3 poles (-52.2385, 6.7736) (-52.7729, 7.2521) (-53.0343, 7.9022) (-53.024, 8.7218) knots 0 0 0 0 1 1 1 1
  line L422 (-53.024, 8.7218) -> (-52.0577, 8.7218)
  line L423 (-36.3274, 7.125) -> (-31.6713, 12.9593)
  line L424 (-31.6713, 12.9593) -> (-35.9863, 12.9593)
  line L425 (-35.9863, 12.9593) -> (-35.9863, 13.8636)
  line L426 (-35.9863, 13.8636) -> (-30.3484, 13.8636)
  line L427 (-30.3484, 13.8636) -> (-30.3484, 12.9799)
  line L428 (-30.3484, 12.9799) -> (-35.0303, 7.1767)
  line L429 (-35.0303, 7.1767) -> (-30.3484, 7.1767)
  line L430 (-30.3484, 7.1767) -> (-30.3484, 6.2723)
  line L431 (-30.3484, 6.2723) -> (-36.3274, 6.2723)
  line L432 (-36.3274, 6.2723) -> (-36.3274, 7.125)
  line L433 (-20.3552, 13.8636) -> (-18.9238, 7.6883)
  line L434 (-18.9238, 7.6883) -> (-17.2081, 13.8636)
  line L435 (-17.2081, 13.8636) -> (-16.0919, 13.8636)
  line L436 (-16.0919, 13.8636) -> (-14.3762, 7.6883)
  line L437 (-14.3762, 7.6883) -> (-12.9448, 13.8636)
  line L438 (-12.9448, 13.8636) -> (-11.8183, 13.8636)
  line L439 (-11.8183, 13.8636) -> (-13.813, 6.2723)
  line L440 (-13.813, 6.2723) -> (-14.893, 6.2723)
  line L441 (-14.893, 6.2723) -> (-16.6448, 12.5665)
  line L442 (-16.6448, 12.5665) -> (-18.407, 6.2723)
  line L443 (-18.407, 6.2723) -> (-19.487, 6.2723)
  line L444 (-19.487, 6.2723) -> (-21.4714, 13.8636)
  line L445 (-21.4714, 13.8636) -> (-20.3552, 13.8636)
  spline S276 degree 3 poles (-0.0329, 14.0703) (1.3076, 14.0703) (2.2997, 13.6393) (2.9436, 12.7784) knots 0 0 0 0 1 1 1 1
  spline S277 degree 3 poles (2.9436, 12.7784) (3.447, 12.1066) (3.6981, 11.2467) (3.6981, 10.1997) knots 0 0 0 0 1 1 1 1
  spline S278 degree 3 poles (3.6981, 10.1997) (3.6981, 9.066) (3.4108, 8.1244) (2.8351, 7.373) knots 0 0 0 0 1 1 1 1
  spline S279 degree 3 poles (2.8351, 7.373) (2.1602, 6.4914) (1.197, 6.0501) (-0.0536, 6.0501) knots 0 0 0 0 1 1 1 1
  spline S280 degree 3 poles (-0.0536, 6.0501) (-1.2215, 6.0501) (-2.1393, 6.4356) (-2.808, 7.2077) knots 0 0 0 0 1 1 1 1
  spline S281 degree 3 poles (-2.808, 7.2077) (-3.4043, 7.9518) (-3.702, 8.8923) (-3.702, 10.0292) knots 0 0 0 0 1 1 1 1
  spline S282 degree 3 poles (-3.702, 10.0292) (-3.702, 11.0555) (-3.4467, 11.934) (-2.9371, 12.6647) knots 0 0 0 0 1 1 1 1
  spline S283 degree 3 poles (-2.9371, 12.6647) (-2.2829, 13.6021) (-1.3145, 14.0703) (-0.0329, 14.0703) knots 0 0 0 0 1 1 1 1
  spline S284 degree 3 poles (0.0704, 6.97) (0.9768, 6.97) (1.6321, 7.2945) (2.0362, 7.9446) knots 0 0 0 0 1 1 1 1
  spline S285 degree 3 poles (2.0362, 7.9446) (2.4413, 8.5936) (2.6439, 9.3399) (2.6439, 10.1842) knots 0 0 0 0 1 1 1 1
  spline S286 degree 3 poles (2.6439, 10.1842) (2.6439, 11.0762) (2.4103, 11.7945) (1.9432, 12.3392) knots 0 0 0 0 1 1 1 1
  spline S287 degree 3 poles (1.9432, 12.3392) (1.4771, 12.8838) (0.8383, 13.1556) (0.0291, 13.1556) knots 0 0 0 0 1 1 1 1
  spline S288 degree 3 poles (0.0291, 13.1556) (-0.7564, 13.1556) (-1.3972, 12.8859) (-1.8933, 12.3474) knots 0 0 0 0 1 1 1 1
  spline S289 degree 3 poles (-1.8933, 12.3474) (-2.3894, 11.8079) (-2.6374, 11.0131) (-2.6374, 9.962) knots 0 0 0 0 1 1 1 1
  spline S290 degree 3 poles (-2.6374, 9.962) (-2.6374, 9.1218) (-2.4245, 8.4128) (-1.9987, 7.835) knots 0 0 0 0 1 1 1 1
  spline S291 degree 3 poles (-1.9987, 7.835) (-1.5739, 7.2583) (-0.8835, 6.97) (0.0704, 6.97) knots 0 0 0 0 1 1 1 1
  line L446 (0.4838, 15.8687) -> (1.4502, 15.8687)
  line L447 (1.4502, 15.8687) -> (1.4502, 14.7938)
  line L448 (1.4502, 14.7938) -> (0.4838, 14.7938)
  line L449 (0.4838, 14.7938) -> (0.4838, 15.8687)
  line L450 (-1.2215, 15.8687) -> (-0.2551, 15.8687)
  line L451 (-0.2551, 15.8687) -> (-0.2551, 14.7938)
  line L452 (-0.2551, 14.7938) -> (-1.2215, 14.7938)
  line L453 (-1.2215, 14.7938) -> (-1.2215, 15.8687)
  line L454 (16.2379, 13.8636) -> (17.2766, 13.8636)
  line L455 (17.2766, 13.8636) -> (17.2766, 6.2723)
  line L456 (17.2766, 6.2723) -> (16.2379, 6.2723)
  line L457 (16.2379, 6.2723) -> (16.2379, 13.8636)
  spline S292 degree 3 poles (31.2861, 8.7218) (31.3099, 8.2908) (31.4122, 7.9415) (31.591, 7.6728) knots 0 0 0 0 1 1 1 1
  spline S293 degree 3 poles (31.591, 7.6728) (31.932, 7.1694) (32.5336, 6.9183) (33.3945, 6.9183) knots 0 0 0 0 1 1 1 1
  spline S294 degree 3 poles (33.3945, 6.9183) (33.78, 6.9183) (34.1314, 6.9731) (34.4487, 7.0837) knots 0 0 0 0 1 1 1 1
  spline S295 degree 3 poles (34.4487, 7.0837) (35.0616, 7.2976) (35.3685, 7.68) (35.3685, 8.2309) knots 0 0 0 0 1 1 1 1
  spline S296 degree 3 poles (35.3685, 8.2309) (35.3685, 8.6443) (35.2393, 8.9388) (34.981, 9.1145) knots 0 0 0 0 1 1 1 1
  spline S297 degree 3 poles (34.981, 9.1145) (34.7195, 9.2871) (34.3092, 9.437) (33.7511, 9.5641) knots 0 0 0 0 1 1 1 1
  line L458 (33.7511, 9.5641) -> (32.7227, 9.7967)
  spline S298 degree 3 poles (32.7227, 9.7967) (32.0509, 9.9486) (31.5755, 10.115) (31.2964, 10.2979) knots 0 0 0 0 1 1 1 1
  spline S299 degree 3 poles (31.2964, 10.2979) (30.8138, 10.6152) (30.573, 11.0886) (30.573, 11.719) knots 0 0 0 0 1 1 1 1
  spline S300 degree 3 poles (30.573, 11.719) (30.573, 12.4012) (30.8086, 12.9613) (31.2809, 13.3985) knots 0 0 0 0 1 1 1 1
  spline S301 degree 3 poles (31.2809, 13.3985) (31.7532, 13.8357) (32.4209, 14.0548) (33.286, 14.0548) knots 0 0 0 0 1 1 1 1
  spline S302 degree 3 poles (33.286, 14.0548) (34.0818, 14.0548) (34.7577, 13.8626) (35.3148, 13.4781) knots 0 0 0 0 1 1 1 1
  spline S303 degree 3 poles (35.3148, 13.4781) (35.8708, 13.0947) (36.1488, 12.4807) (36.1488, 11.6364) knots 0 0 0 0 1 1 1 1
  line L459 (36.1488, 11.6364) -> (35.1825, 11.6364)
  spline S304 degree 3 poles (35.1825, 11.6364) (35.1308, 12.0425) (35.0202, 12.3547) (34.8518, 12.5717) knots 0 0 0 0 1 1 1 1
  spline S305 degree 3 poles (34.8518, 12.5717) (34.5386, 12.9675) (34.0063, 13.166) (33.255, 13.166) knots 0 0 0 0 1 1 1 1
  spline S306 degree 3 poles (33.255, 13.166) (32.6483, 13.166) (32.2132, 13.0389) (31.9476, 12.7836) knots 0 0 0 0 1 1 1 1
  spline S307 degree 3 poles (31.9476, 12.7836) (31.6819, 12.5283) (31.5496, 12.2327) (31.5496, 11.8947) knots 0 0 0 0 1 1 1 1
  spline S308 degree 3 poles (31.5496, 11.8947) (31.5496, 11.5227) (31.7047, 11.2508) (32.0147, 11.0782) knots 0 0 0 0 1 1 1 1
  spline S309 degree 3 poles (32.0147, 11.0782) (32.2183, 10.9677) (32.6783, 10.8302) (33.3945, 10.6648) knots 0 0 0 0 1 1 1 1
  line L460 (33.3945, 10.6648) -> (34.459, 10.422)
  spline S310 degree 3 poles (34.459, 10.422) (34.9727, 10.3052) (35.3685, 10.145) (35.6476, 9.9414) knots 0 0 0 0 1 1 1 1
  spline S311 degree 3 poles (35.6476, 9.9414) (36.1302, 9.5869) (36.3711, 9.0711) (36.3711, 8.3962) knots 0 0 0 0 1 1 1 1
  spline S312 degree 3 poles (36.3711, 8.3962) (36.3711, 7.556) (36.0651, 6.9545) (35.4533, 6.5927) knots 0 0 0 0 1 1 1 1
  spline S313 degree 3 poles (35.4533, 6.5927) (34.8425, 6.231) (34.1314, 6.0501) (33.3221, 6.0501) knots 0 0 0 0 1 1 1 1
  spline S314 degree 3 poles (33.3221, 6.0501) (32.3785, 6.0501) (31.6396, 6.2909) (31.1052, 6.7736) knots 0 0 0 0 1 1 1 1
  spline S315 degree 3 poles (31.1052, 6.7736) (30.5709, 7.2521) (30.3094, 7.9022) (30.3197, 8.7218) knots 0 0 0 0 1 1 1 1
  line L461 (30.3197, 8.7218) -> (31.2861, 8.7218)
  spline S316 degree 3 poles (49.9051, 7.1508) (50.2534, 7.1508) (50.5387, 7.187) (50.7629, 7.2594) knots 0 0 0 0 1 1 1 1
  spline S317 degree 3 poles (50.7629, 7.2594) (51.1629, 7.3937) (51.4895, 7.6521) (51.7448, 8.0345) knots 0 0 0 0 1 1 1 1
  spline S318 degree 3 poles (51.7448, 8.0345) (51.9484, 8.3415) (52.0941, 8.7342) (52.184, 9.2127) knots 0 0 0 0 1 1 1 1
  spline S319 degree 3 poles (52.184, 9.2127) (52.2357, 9.499) (52.2616, 9.7636) (52.2616, 10.0085) knots 0 0 0 0 1 1 1 1
  spline S320 degree 3 poles (52.2616, 10.0085) (52.2616, 10.9491) (52.0745, 11.6798) (51.7014, 12.1996) knots 0 0 0 0 1 1 1 1
  spline S321 degree 3 poles (51.7014, 12.1996) (51.3272, 12.7195) (50.7247, 12.9799) (49.8948, 12.9799) knots 0 0 0 0 1 1 1 1
  line L462 (49.8948, 12.9799) -> (48.0706, 12.9799)
  line L463 (48.0706, 12.9799) -> (48.0706, 7.1508)
  line L464 (48.0706, 7.1508) -> (49.9051, 7.1508)
  line L465 (47.0371, 13.8636) -> (50.1118, 13.8636)
  spline S322 degree 3 poles (50.1118, 13.8636) (51.1557, 13.8636) (51.9649, 13.4936) (52.5406, 12.7526) knots 0 0 0 0 1 1 1 1
  spline S323 degree 3 poles (52.5406, 12.7526) (53.0543, 12.0839) (53.3106, 11.2281) (53.3106, 10.1842) knots 0 0 0 0 1 1 1 1
  spline S324 degree 3 poles (53.3106, 10.1842) (53.3106, 9.3781) (53.1587, 8.6495) (52.8558, 7.9983) knots 0 0 0 0 1 1 1 1
  spline S325 degree 3 poles (52.8558, 7.9983) (52.3215, 6.848) (51.4037, 6.2723) (50.1015, 6.2723) knots 0 0 0 0 1 1 1 1
  line L466 (50.1015, 6.2723) -> (47.0371, 6.2723)
  line L467 (47.0371, 6.2723) -> (47.0371, 13.8636)
  spline S326 degree 3 poles (67.1888, 10.3858) (67.6715, 10.3858) (68.0528, 10.4819) (68.3329, 10.6752) knots 0 0 0 0 1 1 1 1
  spline S327 degree 3 poles (68.3329, 10.6752) (68.614, 10.8684) (68.7546, 11.2157) (68.7546, 11.719) knots 0 0 0 0 1 1 1 1
  spline S328 degree 3 poles (68.7546, 11.719) (68.7546, 12.2596) (68.5582, 12.6285) (68.1655, 12.8249) knots 0 0 0 0 1 1 1 1
  spline S329 degree 3 poles (68.1655, 12.8249) (67.9557, 12.9283) (67.6746, 12.9799) (67.3232, 12.9799) knots 0 0 0 0 1 1 1 1
  line L468 (67.3232, 12.9799) -> (64.8117, 12.9799)
  line L469 (64.8117, 12.9799) -> (64.8117, 10.3858)
  line L470 (64.8117, 10.3858) -> (67.1888, 10.3858)
  line L471 (63.7833, 13.8636) -> (67.2973, 13.8636)
  spline S330 degree 3 poles (67.2973, 13.8636) (67.8761, 13.8636) (68.3536, 13.7789) (68.7288, 13.6104) knots 0 0 0 0 1 1 1 1
  spline S331 degree 3 poles (68.7288, 13.6104) (69.4419, 13.2869) (69.7985, 12.6885) (69.7985, 11.8172) knots 0 0 0 0 1 1 1 1
  spline S332 degree 3 poles (69.7985, 11.8172) (69.7985, 11.3625) (69.7044, 10.9904) (69.5174, 10.701) knots 0 0 0 0 1 1 1 1
  spline S333 degree 3 poles (69.5174, 10.701) (69.3292, 10.4116) (69.0667, 10.1791) (68.7288, 10.0034) knots 0 0 0 0 1 1 1 1
  spline S334 degree 3 poles (68.7288, 10.0034) (69.0254, 9.8825) (69.2486, 9.7243) (69.3975, 9.528) knots 0 0 0 0 1 1 1 1
  spline S335 degree 3 poles (69.3975, 9.528) (69.5473, 9.3316) (69.631, 9.0133) (69.6486, 8.5719) knots 0 0 0 0 1 1 1 1
  line L472 (69.6486, 8.5719) -> (69.6848, 7.5539)
  spline S336 degree 3 poles (69.6848, 7.5539) (69.6951, 7.2645) (69.7189, 7.0496) (69.7571, 6.908) knots 0 0 0 0 1 1 1 1
  spline S337 degree 3 poles (69.7571, 6.908) (69.8191, 6.6671) (69.9297, 6.5121) (70.0879, 6.4429) knots 0 0 0 0 1 1 1 1
  line L473 (70.0879, 6.4429) -> (70.0879, 6.2723)
  line L474 (70.0879, 6.2723) -> (68.827, 6.2723)
  spline S338 degree 3 poles (68.827, 6.2723) (68.7928, 6.3375) (68.7649, 6.4222) (68.7443, 6.5256) knots 0 0 0 0 1 1 1 1
  spline S339 degree 3 poles (68.7443, 6.5256) (68.7236, 6.6289) (68.706, 6.8284) (68.6926, 7.125) knots 0 0 0 0 1 1 1 1
  line L475 (68.6926, 7.125) -> (68.6306, 8.3911)